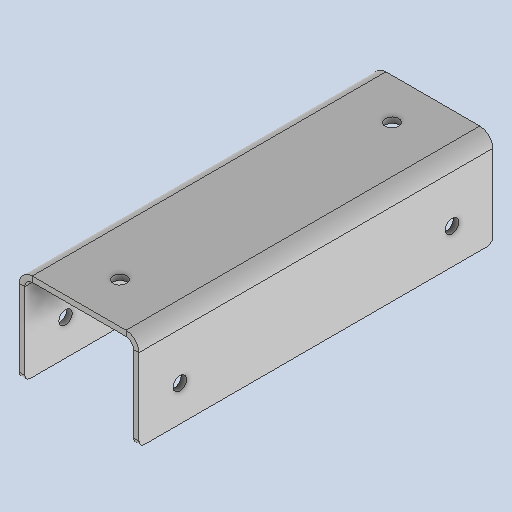
# Autodesk Inventor part: NDM 11.027 bracket 27
Saved by Autodesk Inventor 2025 (Build 290162010, 162A)
## iProperties
Created: 2024-06-12
Part Number: NDM 11.027 bracket 27
Material: Stainless Steel
Document SubType Name: Sheet Metal
Designer: admin
Density: 8 g/cm^3
Flat Pattern Width: 10.6404 cm
Flat Pattern Length: 13 cm
Flat Pattern Area: 138.325 cm^2
Sheet Metal Rule: AISI304 2mm Die16
Sheet Metal Width: 106,404 mm
Sheet Metal Length: 130,000 mm
Sheet Metal Area: 13832,518 mm^2
Appearance: Default
Description: 2mm
Mass: 220.165 g
Surface Area: 286.493 cm^2
Volume: 27.5206 cm^3
Author: admin
Revision Number: 90
Autodesk Inventor part; units mm, degrees
ref_plane "YZ Plane" through (0, 0, 0) normal (1, 0, 0) x (0, 1, 0)
ref_plane "XZ Plane" through (0, 0, 0) normal (0, 1, 0) x (-1, 0, 0)
ref_plane "XY Plane" through (0, 0, 0) normal (0, 0, 1) x (1, 0, 0)
sketch "Sketch1" plane through (0, 0, 0) normal (0, 0, 1) x (1, 0, 0)
  line L0 (-20, 0) -> (20, 0)
  line L1 (20, 0) -> (20, -130)
  line L2 (20, -130) -> (-20, -130)
  line L3 (-20, -130) -> (-20, 0)
  point P0 (0, 0)
  point P1 (0, 0)
  dimension "d0" = 40
  dimension "d1" = 130
  measures "d0" distance of L1.end L2.end
  measures "d1" distance of L0.end L1.end
extrude "Plate1" add sketch "Sketch1" along normal blind 2
sketch "Sketch2" plane through (20, -130, 0) normal (1, 0, 0) x (0, 1, 0)
  line L0 (130, 0) -> (0, 0)
  line L1 (0, 0) -> (0, -33)
  line L2 (0, -33) -> (130, -33)
  line L3 (130, -33) -> (130, 0)
  constraints: 6 end point, 1 horizontal, 1 perpendicular, 1 vertical
edge flange "Flange1" height 35 angle 90 thickness 2 bend radius 2.75 thickness toward (1, 0, 0) relief round relief width 2 relief depth 1 corner gap 2.75 corner form 0 edges at (20, -65, 0) (-20, -65, 0) wall of the first edge with corners at (20, 0, 0) (20, -130, 0) (20, -130, -33) (20, 0, -33)
bend "Bend1"
corner "Corner1"
sketch "Sketch3" plane through (0, 0, 0) normal (1, 0, 0) x (0, 1, 0)
  line L0 (0, -33) -> (-130, -33) projected
  line L1 (-115, -20) -> (-115, -20) construction
  line L2 (-117.5, -20) -> (-117.5, -20)
  line L3 (-112.5, -20) -> (-112.5, -20)
  arc A0 (-112.5, -20) -> (-117.5, -20) centre (-115, -20) ccw
  arc A1 (-117.5, -20) -> (-112.5, -20) centre (-115, -20) ccw
  line L4 (-130, -2.75) -> (-130, -33) projected
  point P0 (0, 0)
  point P1 (-115, -20)
  dimension "d14" = 0
  dimension "d15" = 13
  dimension "d17" = 2.5
  dimension "d18" = 15
  constraints: 8 end point, 4 point on circle, 4 tangent, 2 centre point, 1 midpoint, 1 parallel, 1 vertical
  measures "d14" distance of L1.start L1.end
  measures "d15" distance from line of L0 L1.start
  measures "d17" radius of A1
  measures "d18" distance from line of L4 point (-115, -20)
extrude "Extrusion1" cut sketch "Sketch3" along normal through all both and the other way through all
sketch "Sketch6" plane through (0, 0, 2) normal (0, 0, 1) x (1, 0, 0)
  line L0 (-17.25, 0) -> (17.25, 0) projected
  circle A0 centre (0, -115) radius 2.5
  line L1 (22, -112.5) -> (22, -117.5) projected
  point P0 (0, 0)
  point P1 (0, 0)
  point P2 (22, -115)
  dimension "d27" = 5
  constraints: 2 midpoint, 1 centre point, 1 horizontal alignment, 1 vertical alignment
  measures "d27" diameter of A0
extrude "Extrusion3" cut sketch "Sketch6" against normal blind 10
fillet "Fillet1" radius 2 4 edges at (21, 0, -33) (-21, 0, -33) (21, -130, -33) (-21, -130, -33)
pattern_linear "Rectangular Pattern2" count 2 spacing 100 along (0, 1, 0) of "Extrusion1", "Extrusion3"
equation "\"d2\" = Thickness"
equation "\"d3\" = BendReliefWidth"
equation "\"d4\" = BendReliefDepth"
equation "\"d5\" = MinimumRemnant"
equation "\"d6\" = TransitionRadius"
equation "\"d9\" = BendRadius"
equation "\"d10\" = CornerReliefSize"
equation "\"d11\" = GapSize"
equation "\"d12\" = JacobiRadiusSize"
equation "\"BendReliefWidth\" = Thickness"
equation "\"BendReliefDepth\" = 0.5 * Thickness"
equation "\"CornerReliefSize\" = 4 * Thickness"
equation "\"MinimumRemnant\" = 2 * Thickness"
equation "\"TransitionRadius\" = BendRadius"
equation "\"JacobiRadiusSize\" = BendRadius"
equation "\"GapSize\" = Thickness"
equation "\"Thickness\" = 2"
equation "\"BendRadius\" = 2.75"
body "Solid1"
